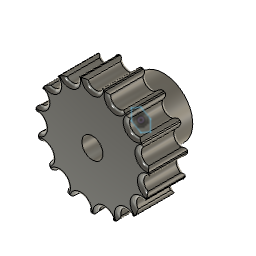
bending_tool_screw_head v3 (Autodesk Fusion 360 design; units mm, degrees)
Autodesk Fusion 360 part; units mm, degrees
note: some values were not read from the file. Set by a fixed rule: which face or edge a step refers to.
sketch "Skizze1" plane through (0, 0, 0) normal (0, 1, 0) x (1, 0, 0)
  circle A0 centre (0, 0) radius 17.5
  line L0 (0, 22.5904) -> (0, -26) construction
  circle A1 centre (0, -17.5) radius 2.5
  circle A2 centre (7.1179, -15.987) radius 2.5
  circle A3 centre (13.005, -11.7098) radius 2.5
  circle A4 centre (16.6435, -5.4078) radius 2.5
  circle A5 centre (17.4041, 1.8292) radius 2.5
  circle A6 centre (15.1554, 8.75) radius 2.5
  circle A7 centre (10.2862, 14.1578) radius 2.5
  circle A8 centre (3.6385, 17.1176) radius 2.5
  circle A9 centre (-3.6385, 17.1176) radius 2.5
  circle A10 centre (-10.2862, 14.1578) radius 2.5
  circle A11 centre (-15.1554, 8.75) radius 2.5
  circle A12 centre (-17.4041, 1.8292) radius 2.5
  circle A13 centre (-16.6435, -5.4078) radius 2.5
  circle A14 centre (-13.005, -11.7098) radius 2.5
  circle A15 centre (-7.1179, -15.987) radius 2.5
  circle A16 centre (0, 0) radius 1.6
  circle A17 centre (0, 0) radius 3.25
  circle A18 centre (0, 0) radius 9
  dimension "d1" = 35
  dimension "d2" = 5
  dimension "d4" = 360
  dimension "d13" = 3.2
  dimension "d14" = 6.5
  dimension "d15" = 18
  constraint coincident A0.centre A16.centre
  constraint vertical L0
  constraint coincident A0.centre L0
  constraint coincident L0 A1.centre
  constraint coincident A0 A1.centre
  constraint concentric A0 A16
  constraint concentric A16 A17
  measures "d1" diameter of A0
  measures "d2" diameter of A1
  measures "d13" diameter of A16
  measures "d14" diameter of A17
  measures "d15" diameter of A18
extrude "Extrusion1" add sketch "Skizze1" along normal blind 12 contours A0 A1 A2 A3 A4 A5 A6 A7 A8 A9 A10 A11 A12 A13 A14 A15 | A17 | A18
fillet "Abrundung2" radius 1 22 faces at (5.9593, 8, -16.1882) (12.1158, 8, -12.4541) (13.8542, 4, -6.6153) (17.3623, 8, 0.6704) (15.5885, 8, 7.6743) (-1.1458, 8, -17.309) (-1.1413, 8, -16.9984) (-7.7889, 4, -14.2738) (-12.1194, 4, -12.4579) (-13.1659, 8, -10.2639) (-15.4422, 8, -6.2665) (-15.909, 8, -3.8329) (-17.3657, 4, 0.6705) (-17.1308, 8, 2.9557) (-15.5899, 4, 7.6749) (-10.5815, 8, 11.096) (-11.1316, 4, 13.3652) (-9.1972, 8, 14.5991) (-4.6198, 8, 16.0835) (2.4816, 4, 17.1971) (9.2617, 4, 14.701) (11.1194, 8, 13.3513)
extrude "Extrusion2" add sketch "Skizze1" along normal blind 22 contours A17 | A18
extrude "Extrusion3" cut sketch "Skizze1" along normal blind 10 contours A17
chamfer "Fase2" distance 1.6 angle 45 1 edges at (-1.4917, 10, -0.5786)
ref_plane "Arbeitsebene1" through (0, 15, 0) normal (0, 1, 0) x (0, 0, 1)
sketch "Skizze2" plane through (0, 15, 0) normal (0, 1, 0) x (1, 0, 0)
  line L0 (2.95, 1.7032) -> (0, 3.4064)
  line L1 (0, 3.4064) -> (-2.95, 1.7032)
  line L2 (-2.95, 1.7032) -> (-2.95, -1.7032)
  line L3 (-2.95, -1.7032) -> (0, -3.4064)
  line L4 (0, -3.4064) -> (2.95, -1.7032)
  line L5 (2.95, -1.7032) -> (2.95, 1.7032)
  dimension "d22" = 5.9
  measures "d22" distance of L2 L5
extrude "Extrusion4" cut sketch "Skizze2" along normal blind 2.8
